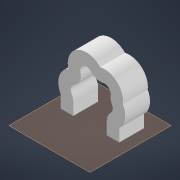
# Autodesk Inventor part: string2
Saved by Autodesk Inventor 2022 (Build 260153000, 153)
## iProperties
Created: 2023-02-08
Part Number: string2
Material: Generic
Document SubType Name: Modeling
Designer: erwin
Density: 1 g/cm^3
Appearance: Default
Author: erwin
Autodesk Inventor part; units mm, degrees
ref_plane "YZ Plane" through (0, 0, 0) normal (1, 0, 0) x (0, 1, 0)
ref_plane "XY Plane" through (0, 0, 0) normal (0, 0, 1) x (1, 0, 0)
sketch "Sketch1" plane through (0, 0, 0) normal (0, 0, 1) x (1, 0, 0)
  line L0 (0.85, 11.55) -> (0.85, -11.55) construction
  arc A0 (0.85, 11.55) -> (-0.85, 11.55) centre (0, 11.55) ccw construction
  line L1 (-0.85, -11.55) -> (-0.85, 11.55) construction
  arc A1 (-0.85, -11.55) -> (0.85, -11.55) centre (0, -11.55) ccw construction
  line L2 (-2.85, 11.55) -> (-2.85, -6.75) construction
  arc A2 (-2.85, 11.55) -> (-4.55, 11.55) centre (-3.7, 11.55) ccw construction
  line L3 (-4.55, -6.75) -> (-4.55, 11.55) construction
  arc A3 (-4.55, -6.75) -> (-2.85, -6.75) centre (-3.7, -6.75) ccw construction
  line L4 (0, 12.4) -> (0, 13.4)
  line L5 (-3.7, 12.4) -> (-3.7, 13.4)
  arc A4 (0.7872, 14.3771) -> (0, 13.4) centre (1, 13.4) ccw
  arc A5 (0.7872, 14.3771) -> (1.3256, 16.0142) centre (0.5744, 15.3542) ccw
  arc A6 (1.1707, 17.0972) -> (1.3256, 16.0142) centre (2.0769, 16.6743) ccw
  arc A7 (1.1707, 17.0972) -> (-0.1098, 18.4474) centre (0.2645, 17.5201) ccw
  arc A8 (-1.1733, 18.65) -> (-0.1098, 18.4474) centre (-0.4842, 19.3746) ccw
  arc A9 (-3.7, 13.4) -> (-4.3417, 14.3336) centre (-4.7, 13.4) ccw
  arc A10 (-3.8648, 16.2602) -> (-4.3417, 14.3336) centre (-3.9835, 15.2672) ccw
  arc A11 (-3.8648, 16.2602) -> (-2.8042, 17.5892) centre (-3.746, 17.2531) ccw
  arc A12 (-1.1733, 18.65) -> (-2.8042, 17.5892) centre (-1.8624, 17.9253) ccw
  point P0 (0, 0)
  dimension "d0" = 1
  dimension "d1" = 1
  dimension "d2" = 1
  dimension "d3" = 1
  dimension "d4" = 1
  dimension "d5" = 1
  dimension "d6" = 1
  dimension "d7" = 1
  dimension "d8" = 1
  dimension "d9" = 1
  dimension "d10" = 1
  constraints: 20 point on circle, 10 tangent, 9 centre point, 4 end point, 2 vertical
  measures "d0" distance of L4.start L4.end
  measures "d1" distance of L5.start L5.end
  measures "d2" radius of A12
  measures "d3" radius of A7
  measures "d4" radius of A11
  measures "d5" radius of A10
  measures "d6" radius of A9
  measures "d7" radius of A8
  measures "d8" radius of A6
  measures "d9" radius of A5
  measures "d10" radius of A4
ref_plane "Work Plane1" through (-3.7, 12.4, 0) normal (0, 1, 0) x (-1, 0, 0)
sketch "Sketch2" plane through (-3.7, 12.4, 0) normal (0, 1, 0) x (-1, 0, 0)
  line L0 (-0.5, 0) -> (0.5, 0)
  line L1 (0.5, 0) -> (0.5, -2)
  line L2 (0.5, -2) -> (-0.5, -2)
  line L3 (-0.5, -2) -> (-0.5, 0)
  point P0 (-3.7, 0)
  point P1 (0, 0)
  dimension "d11" = 1
  dimension "d12" = 2
  constraints: 8 end point, 2 parallel, 1 horizontal, 1 midpoint, 1 perpendicular
  measures "d11" distance of L1.end L2.end
  measures "d12" distance of L0.end L1.end
sweep "Sweep1" add profiles "Sketch2" path "Sketch1"
body "Solid1"
